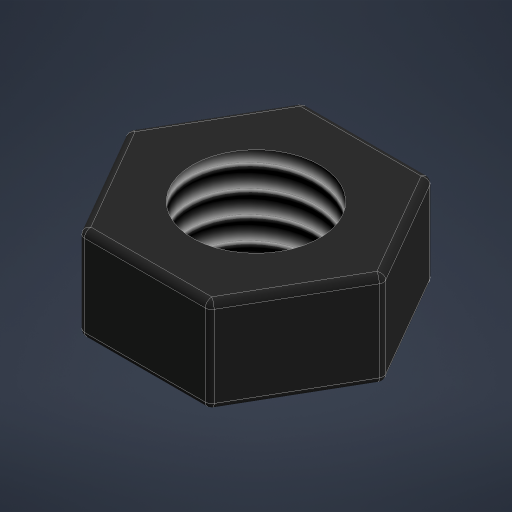
# Autodesk Inventor part: M4 Nut
Saved by Autodesk Inventor 2024 (Build 280153000, 153)
## iProperties
Created: 2024-10-26
Part Number: M4 Nut
Material: Generic
Document SubType Name: Modeling
Designer: jerem
Density: 1 g/cm^3
Appearance: Default
Author: jerem
Autodesk Inventor part; units mm, degrees
ref_plane "YZ Plane" through (0, 0, 0) normal (1, 0, 0) x (0, 1, 0)
ref_plane "XZ Plane" through (0, 0, 0) normal (0, 1, 0) x (-1, 0, 0)
ref_plane "XY Plane" through (0, 0, 0) normal (0, 0, 1) x (1, 0, 0)
sketch "Sketch1" plane through (0, 0, 0) normal (0, 1, 0) x (-1, 0, 0)
  line L0 (3.9837, 0) -> (1.9919, -3.45)
  line L1 (1.9919, -3.45) -> (-1.9919, -3.45)
  line L2 (-1.9919, -3.45) -> (-3.9837, 0)
  line L3 (-3.9837, 0) -> (-1.9919, 3.45)
  line L4 (-1.9919, 3.45) -> (1.9919, 3.45)
  line L5 (1.9919, 3.45) -> (3.9837, 0)
  circle A0 centre (0, 0) radius 1.97
  dimension "d0" = 6.9
  dimension "d1" = 3.94
  constraints: 12 end point, 2 coincident, 1 centre point, 1 horizontal, 13 other
  measures "d0" distance between parallel lines of L4 L1
  measures "d1" diameter of A0
extrude "Extrusion1" add sketch "Sketch1" along normal blind 2.93
fillet "Fillet1" radius 0.2 18 edges at (2.9878, 2.93, 1.725) (0, 2.93, 3.45) (1.9919, 1.465, 3.45) (0, 0, 3.45) (-1.9919, 1.465, 3.45) (2.9878, 0, 1.725) (3.9837, 1.465, 0) (1.9919, 1.465, -3.45) (2.9878, 2.93, -1.725) (2.9878, 0, -1.725) (-1.9919, 1.465, -3.45) (0, 2.93, -3.45) (0, 0, -3.45) (-2.9878, 2.93, 1.725) (-2.9878, 2.93, -1.725) (-3.9837, 1.465, 0) (-2.9878, 0, -1.725) (-2.9878, 0, 1.725)
thread "Thread1" size "M4x0.7" class "6H" standard "ANSI Metric M Profile" full length
body "Solid1"
